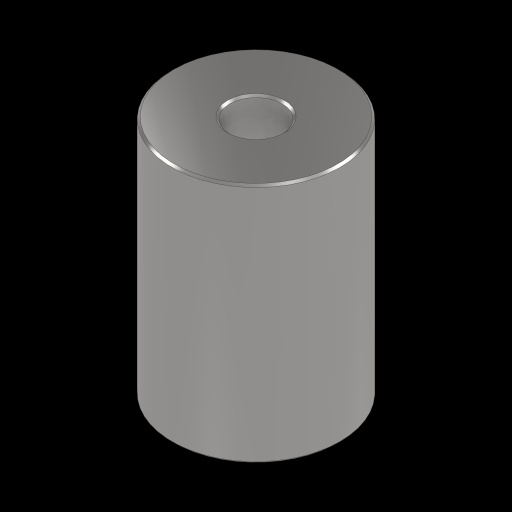
# Autodesk Inventor part: Distanzbuchse wie MISUMI DWSSS-D16-V5-L23
Saved by Autodesk Inventor 2024 (Build 280153000, 153)
## iProperties
Created: 2023-09-21
Part Number: Distanzbuchse wie MISUMI DWSSS-D16-V5-L23
Material: Edelstahl
Document SubType Name: Modeling
Designer: buchmannmartin
Density: 8 g/cm^3
Appearance: Halbpoliert
Author: buchmannmartin
Autodesk Inventor part; units mm, degrees
ref_plane "YZ Plane" through (0, 0, 0) normal (1, 0, 0) x (0, 1, 0)
ref_plane "XZ Plane" through (0, 0, 0) normal (0, 1, 0) x (-1, 0, 0)
ref_plane "XY Plane" through (0, 0, 0) normal (0, 0, 1) x (1, 0, 0)
sketch "Skizze1" plane through (0, 0, 0) normal (0, 0, 1) x (1, 0, 0)
  line L0 (-8, 11.5) -> (-2.5, 11.5)
  line L1 (-2.5, 11.5) -> (-2.5, -11.5)
  line L2 (-2.5, -11.5) -> (-8, -11.5)
  line L3 (-8, -11.5) -> (-8, 11.5)
  line L4 (0, 11.5) -> (0, -11.5) construction
  point P0 (0, 0)
  point P1 (0, 0)
  dimension "d0" = 5
  dimension "d1" = 16
  dimension "d2" = 23
  constraints: 10 end point, 2 parallel, 2 point on line, 1 coincident, 1 horizontal, 1 midpoint, 1 perpendicular, 1 vertical
  measures "d0" diameter of L1 L4
  measures "d1" diameter of L3 L4
  measures "d2" distance of L2.end L0.start
revolve "Umdrehung1" add sketch "Skizze1" angle 360 about axis through (0, 11.5, 0) along (0, -1, 0)
chamfer "Fasen1" distance 0.2 angle 45 4 edges at (8, 11.5, 0) (2.5, 11.5, 0) (8, -11.5, 0) (2.5, -11.5, 0)
